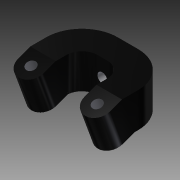
# Autodesk Inventor part: MountB
Saved by Autodesk Inventor 2015 (Build 190159000, 159)
## iProperties
Created: 2017-01-08
Part Number: MountB
Material: Generic
Document SubType Name: Modeling
Designer: Ernest
Density: 1 g/cm^3
Appearance: Default
Mass: 135.561 g
Surface Area: 237.117 cm^2
Volume: 135.561 cm^3
Author: Ernest
Autodesk Inventor part; units mm, degrees
note: some values were not read from the file. Chosen so that the rebuilt part matches the saved one: sketch regions of "Extrusion29".
ref_plane "YZ Plane" through (0, 0, 0) normal (1, 0, 0) x (0, 1, 0)
ref_plane "XZ Plane" through (0, 0, 0) normal (0, 1, 0) x (-1, 0, 0)
sketch "Sketch1" plane through (0, 0, 0) normal (0, 0, 1) x (1, 0, 0)
  circle A0 centre (0, 0) radius 5
  circle A1 centre (65, 0) radius 5
  circle A2 centre (0, 0) radius 12.5
  circle A3 centre (65, 0) radius 12.5
  line L0 (22.5, 9.5) -> (42.5, 9.5)
  line L1 (42.5, 9.5) -> (42.5, -10.5)
  line L2 (42.5, -10.5) -> (22.5, -10.5)
  line L3 (22.5, -10.5) -> (22.5, 9.5)
  line L4 (0, 0) -> (65, 0) construction
  line L5 (32.5, 0) -> (32.5, 30) construction
  line L6 (27.5, 30) -> (37.5, 30)
  line L7 (12.5, 0) -> (12.5, 15)
  line L8 (52.5, 0) -> (52.5, 15)
  arc A4 (27.5, 30) -> (12.5, 15) centre (27.5, 15) ccw
  arc A5 (52.5, 15) -> (37.5, 30) centre (37.5, 15) ccw
  line L9 (-12.5, 0) -> (-12.5, 20)
  line L10 (77.5, 0) -> (77.5, 20)
  line L11 (22.5, 55) -> (42.5, 55)
  arc A6 (22.5, 55) -> (-12.5, 20) centre (22.5, 20) ccw
  arc A7 (77.5, 20) -> (42.5, 55) centre (42.5, 20) ccw
  point P0 (22.5, 30)
  point P1 (42.5, 30)
  dimension "d0" = 10
  dimension "d1" = 10
  dimension "d2" = 65
  dimension "d3" = 25
  dimension "d4" = 25
  dimension "d5" = 22.5
  dimension "d6" = 22.5
  dimension "d7" = 9.5
  dimension "d8" = 10.5
  dimension "d11" = 20
  dimension "d12" = 10
  dimension "d13" = 30
  dimension "d14" = 15
  dimension "d15" = 55
  dimension "d16" = 35
  constraints: 24 end point, 12 point on circle, 12 tangent, 8 centre point, 4 horizontal, 4 point on line, 3 coincident, 3 perpendicular, 3 vertical, 2 equal radius, 2 midpoint, 2 parallel
  measures "d0" diameter of A0
  measures "d1" diameter of A1
  measures "d2" distance of A1.centre point (0, 0)
  measures "d3" diameter of A2
  measures "d4" diameter of A3
  measures "d5" distance from line of L3 point (0, 0)
  measures "d6" distance from line of L1 A1.centre
  measures "d7" distance from line of L0 point (0, 0)
  measures "d8" distance from line of point (0, 0) L2
  measures "d11" distance of point (22.5, 30) point (42.5, 30)
  measures "d12" distance of L5.end point (22.5, 30)
  measures "d13" distance of L5.start L5.end
  measures "d14" radius of A4
  measures "d15" distance from line of L11 L5.start
  measures "d16" radius of A6
extrude "Extrusion1" add sketch "Sketch1" along normal blind 34 contours A0 | A1 | A2 | A2 L9 A6 L11 A7 L10 A3 L8 A5 L6 A4 L7 | A3
ref_plane "Work Plane4" through (42.5, 55, 0) normal (0, 0.3420201, -0.9396926) x (-1, 0, 0)
sketch "Sketch23" plane through (42.5, 55, 0) normal (0, 0.3420201, -0.9396926) x (-1, 0, 0)
  ellipse E0 centre (42.5, -40.0544) end of major axis (30, -40.0544) minor radius 11.7462 (30, -40.0544) -> (55, -40.0544) ccw projected
  line L0 (30, -40.0544) -> (30, -25.959) projected
  ellipse E1 centre (15, -25.959) end of major axis (30, -25.959) minor radius 14.0954 (30, -25.959) -> (15, -11.8636) ccw projected
  line L1 (15, -11.8636) -> (5, -11.8636) projected
  ellipse E2 centre (5, -25.959) end of major axis (20, -25.959) minor radius 14.0954 (5, -11.8636) -> (-10, -25.959) ccw projected
  line L2 (-10, -25.959) -> (-10, -40.0544) projected
  ellipse E3 centre (-22.5, -40.0544) end of major axis (-35, -40.0544) minor radius 11.7462 (-35, -40.0544) -> (-10, -40.0544) ccw projected
  line L3 (-35, -40.0544) -> (-35, -21.2606) projected
  ellipse E4 centre (0, -21.2606) end of major axis (-35, -21.2606) minor radius 32.8892 (0, 11.6287) -> (-35, -21.2606) ccw projected
  line L4 (0, 11.6287) -> (20, 11.6287) projected
  ellipse E5 centre (20, -21.2606) end of major axis (55, -21.2606) minor radius 32.8892 (55, -21.2606) -> (20, 11.6287) ccw projected
  line L5 (55, -21.2606) -> (55, -40.0544) projected
  ellipse E6 centre (42.5, -51.6831) end of major axis (30, -51.6831) minor radius 11.7462 (30, -51.6831) -> (55, -51.6831) ccw projected
  line L6 (55, -32.8892) -> (55, -51.6831) projected
  ellipse E7 centre (20, -32.8892) end of major axis (55, -32.8892) minor radius 32.8892 (55, -32.8892) -> (20, 0) ccw projected
  line L7 (0, 0) -> (20, 0) projected
  ellipse E8 centre (0, -32.8892) end of major axis (-35, -32.8892) minor radius 32.8892 (0, 0) -> (-35, -32.8892) ccw projected
  line L8 (-35, -51.6831) -> (-35, -32.8892) projected
  ellipse E9 centre (-22.5, -51.6831) end of major axis (-35, -51.6831) minor radius 11.7462 (-35, -51.6831) -> (-10, -51.6831) ccw projected
  line L9 (-10, -37.5877) -> (-10, -51.6831) projected
  ellipse E10 centre (5, -37.5877) end of major axis (20, -37.5877) minor radius 14.0954 (5, -23.4923) -> (-10, -37.5877) ccw projected
  line L10 (15, -23.4923) -> (5, -23.4923) projected
  ellipse E11 centre (15, -37.5877) end of major axis (30, -37.5877) minor radius 14.0954 (30, -37.5877) -> (15, -23.4923) ccw projected
  line L11 (30, -51.6831) -> (30, -37.5877) projected
  line L12 (0, 0) -> (20, 0) projected
  line L13 (10, 0) -> (10, -36)
  circle A0 centre (-22.5, -48.5) radius 5
  circle A1 centre (42.5, -48.5) radius 5
  circle A2 centre (-22.5, -48.5) radius 12.5
  circle A3 centre (42.5, -48.5) radius 12.5
  line L14 (-35, -36) -> (-10, -36)
  line L15 (-35, -36) -> (-35, -48.5)
  line L16 (-35, -51.6831) -> (-35, -40.0544) projected
  line L17 (-10, -36) -> (-10, -48.5)
  line L18 (-10, -51.6831) -> (-10, -40.0544) projected
  line L19 (30, -36) -> (55, -36)
  line L20 (30, -51.6831) -> (30, -40.0544) projected
  line L21 (30, -48.5) -> (30, -36)
  line L22 (55, -48.5) -> (55, -36)
  dimension "d108" = 36
  dimension "d110" = 10
  dimension "d111" = 10
  dimension "d112" = 12.5
  dimension "d113" = 12.5
  dimension "d114" = 25
  dimension "d115" = 25
  constraints: 14 end point, 8 point on line, 4 centre point, 4 point on circle, 3 tangent, 2 coincident, 2 horizontal, 2 perpendicular, 1 midpoint, 1 vertical, 12 other
  measures "d108" distance of L13.start L13.end
  measures "d110" diameter of A0
  measures "d111" diameter of A1
  measures "d112" vertical distance of L13.end A0.centre
  measures "d113" vertical distance of L13.end A1.centre
  measures "d114" diameter of A2
  measures "d115" diameter of A3
extrude "Extrusion29" add sketch "Sketch23" against normal blind 49.285 contours L0 L19 A3 E0 | E0 A3 L11 | A3 E0 A1 | E0 A1 A3 | L19 L5 E0 A3 | A3 E0 L6 | L2 E3 A2 L14 | L9 A2 E3 | A2 E3 A0 | A2 E3 L3 L14 | A2 E3 A0 | A2 L8 E3
sketch "Sketch24" plane through (42.5, 55, 0) normal (0, 0.3420201, -0.9396926) x (-1, 0, 0)
  circle A0 centre (-22.5, -48.5) radius 5 projected
  arc A1 (-35, -48.5) -> (-10, -48.5) centre (-22.5, -48.5) ccw projected
  line L0 (-10, -48.5) -> (-10, -36) projected
  line L1 (-10, -36) -> (-35, -36) projected
  line L2 (-35, -36) -> (-35, -48.5) projected
  circle A2 centre (42.5, -48.5) radius 5 projected
  arc A3 (30, -48.5) -> (55, -48.5) centre (42.5, -48.5) ccw projected
  line L3 (55, -48.5) -> (55, -36) projected
  line L4 (30, -36) -> (55, -36) projected
  line L5 (30, -36) -> (30, -48.5) projected
  point P0 (42.5, -51.6831)
extrude "Extrusion30" cut sketch "Sketch24" against normal blind 13.103
sketch "Sketch25" plane through (77.5, 20, 34) normal (1, 0, 0) x (0, 0, -1)
  line L0 (1.5704, -20) -> (1.5704, -20) projected
  line L1 (1.5704, -20) -> (4.2752, -27.4316) projected
  line L2 (4.2752, -27.4316) -> (4.2752, -27.4316) projected
  line L3 (4.2752, -27.4316) -> (1.5704, -20) projected
  line L4 (-2.4671, -8.9071) -> (10.0523, -43.304)
  line L5 (10.0523, -43.304) -> (-2.0937, -47.7247)
  line L6 (-2.4671, -8.9071) -> (-14.6131, -13.3279)
  line L7 (-2.0937, -47.7247) -> (-14.6131, -13.3279)
  point P0 (34, -20)
  constraints: 8 end point, 3 perpendicular, 2 point on line
extrude "Extrusion31" cut sketch "Sketch25" against normal blind 100
sketch "Sketch26" plane through (42.5, 50.5185, 12.3128) normal (0, 0.3420201, -0.9396926) x (-1, 0, 0)
  circle A0 centre (-22.5, -48.5) radius 5 projected
  arc A1 (-35, -48.5) -> (-10, -48.5) centre (-22.5, -48.5) ccw projected
  line L0 (-10, -36.0002) -> (-10, -48.5) projected
  line L1 (-10, -36) -> (-10, -36.0002) projected
  line L2 (-35, -36) -> (-10, -36) projected
  line L3 (-35, -48.5) -> (-35, -36) projected
  circle A2 centre (42.5, -48.5) radius 5 projected
  arc A3 (30, -48.5) -> (55, -48.5) centre (42.5, -48.5) ccw projected
  line L4 (55, -36) -> (55, -48.5) projected
  line L5 (30, -36) -> (55, -36) projected
  line L6 (30, -36.0002) -> (30, -36) projected
  line L7 (30, -48.5) -> (30, -36.0002) projected
  line L8 (-35, -36) -> (-43.7615, -36)
  line L9 (-43.7615, -36) -> (-43.7615, -67.4165)
  line L10 (-43.7615, -67.4165) -> (-2.78, -67.4165)
  line L11 (-2.78, -67.4165) -> (-2.78, -36)
  line L12 (-2.78, -36) -> (-10, -36)
  line L13 (30, -36.0002) -> (23.7348, -36)
  line L14 (23.7348, -36) -> (23.7338, -67.4165)
  line L15 (23.7338, -67.4165) -> (61.4136, -67.4165)
  line L16 (61.4136, -67.4165) -> (61.4136, -36.0012)
  line L17 (61.4136, -36.0012) -> (55, -36)
  point P0 (42.5, -51.6831)
  constraints: 20 end point, 6 perpendicular, 5 point on line, 1 horizontal
extrude "Extrusion32" cut sketch "Sketch26" against normal blind 100 contours A0 | A1 L0 L12 L11 L10 L9 L8 L3 | A2 | A3 L4 L17 L16 L15 L14 L13 L7
sketch "Sketch27" plane through (22.5, 55, 0) normal (0, 1, 0) x (1, 0, 0)
  circle A0 centre (10, -17) radius 5
  line L0 (20, 0) -> (0, 0) projected
  line L1 (0, 0) -> (0, -34) projected
  line L2 (20, -34) -> (0, -34) projected
  line L3 (20, 0) -> (20, -34) projected
  point P0 (-22.5, 0)
  dimension "d124" = 10
  dimension "d125" = 20
  dimension "d126" = 34
  dimension "d127" = 10
  dimension "d128" = 17
  constraints: 1 centre point
  measures "d124" diameter of A0
  measures "d125" distance of L0.start L0.end
  measures "d126" distance of L0.end L1.end
  measures "d127" distance from line of L1 A0.centre
  measures "d128" distance from line of L0 A0.centre
extrude "Extrusion33" cut sketch "Sketch27" against normal blind 100 contours A0
sketch "Sketch28" plane through (42.5, 38.1435, 46.3128) normal (0, -0.3420201, 0.9396926) x (1, 0, 0)
  circle A0 centre (-42.5, -48.5) radius 5 projected
  line L0 (-55, -48.5) -> (-55, -36) projected
  arc A1 (-55, -48.5) -> (-30, -48.5) centre (-42.5, -48.5) ccw projected
  line L1 (-30, -36) -> (-30, -48.5) projected
  line L2 (-55, -36) -> (-30, -36) projected
  circle A2 centre (22.5, -48.5) radius 5 projected
  line L3 (35, -36) -> (35, -48.5) projected
  line L4 (35, -36) -> (10, -36) projected
  line L5 (10, -48.5) -> (10, -36) projected
  arc A3 (10, -48.5) -> (35, -48.5) centre (22.5, -48.5) ccw projected
  circle A4 centre (22.5, -48.5) radius 4.75
  circle A5 centre (22.5, -48.5) radius 5
  circle A6 centre (-42.5, -48.5) radius 5
  circle A7 centre (-42.5, -48.5) radius 4.75
  point P0 (-42.5, -51.6831)
  dimension "d131" = 9.5
  dimension "d132" = 9.5
  constraints: 4 centre point, 4 coincident, 1 concentric
  measures "d131" diameter of A4
  measures "d132" diameter of A7
extrude "Extrusion34" add sketch "Sketch28" against normal up to surface (36.182 mm away) contours A0 | A2
sketch "Sketch29" plane through (22.5, 55, 0) normal (0, 1, 0) x (1, 0, 0)
  circle A0 centre (10, -17) radius 5 projected
  line L0 (20, 0) -> (0, 0) projected
  line L1 (0, 0) -> (0, -34) projected
  line L2 (20, -34) -> (0, -34) projected
  line L3 (20, 0) -> (20, -34) projected
  circle A1 centre (10, -17) radius 4.75
  point P0 (-22.5, 0)
  dimension "d135" = 9.5
  constraints: 1 centre point, 1 coincident
  measures "d135" diameter of A1
extrude "Extrusion35" add sketch "Sketch29" against normal up to surface (25 mm away) contours A0
equation "\"d12\" = 0.5 * d11"
equation "\"d15\" = d13 + d3"
body "Solid1"
